Autodesk Inventor part; units mm, degrees
(part 2 of 4)
  spline S206 degree 2 poles (-53.4859, 25.985) (-53.3352, 26.0295) (-53.0931, 26.0739) (-52.9227, 26.0739) knots 0 0 0 1 2 2 2
  line L241 (-55.6274, 24.1399) -> (-55.6076, 24.1399)
  spline S207 degree 2 poles (-55.6076, 24.1399) (-55.5632, 24.1276) (-55.4668, 24.1226) (-55.4001, 24.1226) knots 0 0 0 1 2 2 2
  spline S208 degree 2 poles (-55.4001, 24.1226) (-55.2445, 24.1226) (-54.9382, 24.2585) (-54.7999, 24.3919) knots 0 0 0 1 2 2 2
  line L242 (-54.7999, 24.3919) -> (-54.7999, 26.0147)
  line L243 (-54.7999, 26.0147) -> (-54.4146, 26.0147)
  line L244 (-54.4146, 26.0147) -> (-54.4146, 23.7274)
  line L245 (-54.4146, 23.7274) -> (-54.7999, 23.7274)
  line L246 (-54.7999, 23.7274) -> (-54.7999, 24.0683)
  spline S209 degree 2 poles (-54.7999, 24.0683) (-55.0099, 23.8806) (-55.3236, 23.7274) (-55.4718, 23.7274) knots 0 0 0 1 2 2 2
  spline S210 degree 2 poles (-55.4718, 23.7274) (-55.5311, 23.7274) (-55.5903, 23.7324) (-55.6274, 23.7398) knots 0 0 0 1 2 2 2
  line L247 (-55.6274, 23.7398) -> (-55.6274, 24.1399)
  spline S211 degree 2 poles (-57.8059, 24.871) (-57.8059, 25.449) (-57.2502, 26.0789) (-56.7858, 26.0789) knots 0 0 0 1 2 2 2
  spline S212 degree 2 poles (-56.7858, 26.0789) (-56.3091, 26.0789) (-55.7632, 25.4293) (-55.7632, 24.871) knots 0 0 0 1 2 2 2
  spline S213 degree 2 poles (-55.7632, 24.871) (-55.7632, 24.298) (-56.3264, 23.6632) (-56.7858, 23.6632) knots 0 0 0 1 2 2 2
  spline S214 degree 2 poles (-56.7858, 23.6632) (-57.2502, 23.6632) (-57.8059, 24.2955) (-57.8059, 24.871) knots 0 0 0 1 2 2 2
  spline S215 degree 2 poles (-57.4083, 24.871) (-57.4083, 24.4264) (-57.0847, 23.9942) (-56.7858, 23.9942) knots 0 0 0 1 2 2 2
  spline S216 degree 2 poles (-56.7858, 23.9942) (-56.4869, 23.9942) (-56.1609, 24.4264) (-56.1609, 24.871) knots 0 0 0 1 2 2 2
  spline S217 degree 2 poles (-56.1609, 24.871) (-56.1609, 25.3033) (-56.4869, 25.7479) (-56.7858, 25.7479) knots 0 0 0 1 2 2 2
  spline S218 degree 2 poles (-56.7858, 25.7479) (-57.0822, 25.7479) (-57.4083, 25.3107) (-57.4083, 24.871) knots 0 0 0 1 2 2 2
  line L248 (-59.9795, 26.0147) -> (-59.5942, 26.0147)
  line L249 (-59.5942, 26.0147) -> (-59.5942, 25.7627)
  spline S219 degree 2 poles (-59.5942, 25.7627) (-59.4164, 25.9183) (-59.0978, 26.0789) (-58.9002, 26.0789) knots 0 0 0 1 2 2 2
  spline S220 degree 2 poles (-58.9002, 26.0789) (-58.752, 26.0789) (-58.4877, 25.9801) (-58.3913, 25.8739) knots 0 0 0 1 2 2 2
  spline S221 degree 2 poles (-58.3913, 25.8739) (-58.2925, 25.7677) (-58.1838, 25.4441) (-58.1838, 25.2119) knots 0 0 0 1 2 2 2
  line L250 (-58.1838, 25.2119) -> (-58.1838, 23.7274)
  line L251 (-58.1838, 23.7274) -> (-58.5692, 23.7274)
  line L252 (-58.5692, 23.7274) -> (-58.5692, 25.0316)
  spline S222 degree 2 poles (-58.5692, 25.0316) (-58.5692, 25.2144) (-58.5963, 25.454) (-58.6433, 25.5429) knots 0 0 0 1 2 2 2
  spline S223 degree 2 poles (-58.6433, 25.5429) (-58.6902, 25.6318) (-58.8508, 25.7133) (-59.0014, 25.7133) knots 0 0 0 1 2 2 2
  spline S224 degree 2 poles (-59.0014, 25.7133) (-59.1422, 25.7133) (-59.4608, 25.5528) (-59.5942, 25.4367) knots 0 0 0 1 2 2 2
  line L253 (-59.5942, 25.4367) -> (-59.5942, 23.7274)
  line L254 (-59.5942, 23.7274) -> (-59.9795, 23.7274)
  line L255 (-59.9795, 23.7274) -> (-59.9795, 26.0147)
  line L256 (-62.3335, 26.0147) -> (-61.9482, 26.0147)
  line L257 (-61.9482, 26.0147) -> (-61.9482, 24.7105)
  spline S225 degree 2 poles (-61.9482, 24.7105) (-61.9482, 24.5524) (-61.9185, 24.2807) (-61.8741, 24.1992) knots 0 0 0 1 2 2 2
  spline S226 degree 2 poles (-61.8741, 24.1992) (-61.8271, 24.1127) (-61.6592, 24.0288) (-61.5159, 24.0288) knots 0 0 0 1 2 2 2
  spline S227 degree 2 poles (-61.5159, 24.0288) (-61.3726, 24.0288) (-61.0688, 24.1819) (-60.9231, 24.3054) knots 0 0 0 1 2 2 2
  line L258 (-60.9231, 24.3054) -> (-60.9231, 26.0147)
  line L259 (-60.9231, 26.0147) -> (-60.5378, 26.0147)
  line L260 (-60.5378, 26.0147) -> (-60.5378, 23.7274)
  line L261 (-60.5378, 23.7274) -> (-60.9231, 23.7274)
  line L262 (-60.9231, 23.7274) -> (-60.9231, 23.9818)
  spline S228 degree 2 poles (-60.9231, 23.9818) (-61.096, 23.8262) (-61.4294, 23.6632) (-61.6172, 23.6632) knots 0 0 0 1 2 2 2
  spline S229 degree 2 poles (-61.6172, 23.6632) (-61.9531, 23.6632) (-62.3335, 24.1078) (-62.3335, 24.5302) knots 0 0 0 1 2 2 2
  line L263 (-62.3335, 24.5302) -> (-62.3335, 26.0147)
  line L264 (-64.6331, 26.0147) -> (-64.2477, 26.0147)
  line L265 (-64.2477, 26.0147) -> (-64.2477, 25.7825)
  spline S230 degree 2 poles (-64.2477, 25.7825) (-64.1588, 25.8566) (-64.0279, 25.9554) (-63.939, 25.9974) knots 0 0 0 1 2 2 2
  spline S231 degree 2 poles (-63.939, 25.9974) (-63.8575, 26.0369) (-63.6821, 26.0789) (-63.566, 26.0789) knots 0 0 0 1 2 2 2
  spline S232 degree 2 poles (-63.566, 26.0789) (-63.3783, 26.0789) (-63.0621, 25.9233) (-62.951, 25.7726) knots 0 0 0 1 2 2 2
  spline S233 degree 2 poles (-62.951, 25.7726) (-62.8398, 25.6219) (-62.7163, 25.1773) (-62.7163, 24.8883) knots 0 0 0 1 2 2 2
  spline S234 degree 2 poles (-62.7163, 24.8883) (-62.7163, 24.587) (-62.8719, 24.1473) (-63.0078, 23.9818) knots 0 0 0 1 2 2 2
  spline S235 degree 2 poles (-63.0078, 23.9818) (-63.1338, 23.8336) (-63.487, 23.6632) (-63.6821, 23.6632) knots 0 0 0 1 2 2 2
  spline S236 degree 2 poles (-63.6821, 23.6632) (-63.8525, 23.6632) (-64.1069, 23.7398) (-64.2477, 23.8188) knots 0 0 0 1 2 2 2
  line L266 (-64.2477, 23.8188) -> (-64.2477, 22.8308)
  line L267 (-64.2477, 22.8308) -> (-64.6331, 22.8308)
  line L268 (-64.6331, 22.8308) -> (-64.6331, 26.0147)
  line L269 (-64.2477, 25.4589) -> (-64.2477, 24.1374)
  spline S237 degree 2 poles (-64.2477, 24.1374) (-64.1045, 24.0683) (-63.8772, 24.0164) (-63.7463, 24.0164) knots 0 0 0 1 2 2 2
  spline S238 degree 2 poles (-63.7463, 24.0164) (-63.4499, 24.0164) (-63.114, 24.461) (-63.114, 24.8809) knots 0 0 0 1 2 2 2
  spline S239 degree 2 poles (-63.114, 24.8809) (-63.114, 25.286) (-63.3709, 25.7133) (-63.6549, 25.7133) knots 0 0 0 1 2 2 2
  spline S240 degree 2 poles (-63.6549, 25.7133) (-63.8056, 25.7133) (-64.1119, 25.575) (-64.2477, 25.4589) knots 0 0 0 1 2 2 2
  spline S241 degree 2 poles (51.1339, 19.6673) (51.5277, 19.8947) (52.3044, 19.9435) (52.6446, 19.8089) knots 0 0 0 1 2 2 2
  spline S242 degree 2 poles (52.6446, 19.8089) (53.0488, 19.6427) (53.6387, 19.0757) (53.9502, 18.5363) knots 0 0 0 1 2 2 2
  line L270 (53.9502, 18.5363) -> (54.8251, 17.0208)
  line L271 (54.8251, 17.0208) -> (49.5424, 13.9708)
  line L272 (49.5424, 13.9708) -> (48.7342, 15.3707)
  spline S243 degree 2 poles (48.7342, 15.3707) (48.4079, 15.9358) (48.1544, 16.5429) (48.1474, 16.8814) knots 0 0 0 1 2 2 2
  spline S244 degree 2 poles (48.1474, 16.8814) (48.1316, 17.2547) (48.4732, 17.8001) (48.8071, 17.9929) knots 0 0 0 1 2 2 2
  spline S245 degree 2 poles (48.8071, 17.9929) (49.1795, 18.2079) (49.9977, 18.1551) (50.3649, 17.9048) knots 0 0 0 1 2 2 2
  line L273 (50.3649, 17.9048) -> (50.3906, 17.9196)
  spline S246 degree 2 poles (50.3906, 17.9196) (50.2471, 18.4646) (50.6287, 19.3756) (51.1339, 19.6673) knots 0 0 0 1 2 2 2
  spline S247 degree 2 poles (51.5865, 18.9525) (51.2868, 18.7795) (51.0004, 18.3858) (51.0117, 18.0499) knots 0 0 0 1 2 2 2
  spline S248 degree 2 poles (51.0117, 18.0499) (51.0225, 17.8335) (51.1985, 17.41) (51.4086, 17.0461) knots 0 0 0 1 2 2 2
  line L274 (51.4086, 17.0461) -> (51.8683, 16.2498)
  line L275 (51.8683, 16.2498) -> (53.8204, 17.3769)
  line L276 (53.8204, 17.3769) -> (53.4917, 17.9463)
  spline S249 degree 2 poles (53.4917, 17.9463) (53.2248, 18.4086) (52.8327, 18.89) (52.577, 19.0164) knots 0 0 0 1 2 2 2
  spline S250 degree 2 poles (52.577, 19.0164) (52.3221, 19.1318) (51.8648, 19.1132) (51.5865, 18.9525) knots 0 0 0 1 2 2 2
  spline S251 degree 2 poles (49.3282, 17.3177) (49.1398, 17.2089) (48.9314, 16.9173) (48.9317, 16.7291) knots 0 0 0 1 2 2 2
  spline S252 degree 2 poles (48.9317, 16.7291) (48.9364, 16.5035) (49.1333, 16.0635) (49.3483, 15.6911) knots 0 0 0 1 2 2 2
  line L277 (49.3483, 15.6911) -> (49.7364, 15.019)
  line L278 (49.7364, 15.019) -> (51.2818, 15.9112)
  line L279 (51.2818, 15.9112) -> (50.8221, 16.7075)
  spline S253 degree 2 poles (50.8221, 16.7075) (50.6318, 17.0371) (50.3828, 17.3101) (50.1794, 17.4153) knots 0 0 0 1 2 2 2
  spline S254 degree 2 poles (50.1794, 17.4153) (49.9828, 17.5186) (49.5765, 17.461) (49.3282, 17.3177) knots 0 0 0 1 2 2 2
  spline S255 degree 2 poles (50.6883, 23.2173) (50.7951, 23.1705) (51.1674, 23.0201) (51.3057, 22.9288) knots 0 0 0 1 2 2 2
  spline S256 degree 2 poles (51.3057, 22.9288) (51.5013, 22.8076) (51.79, 22.5348) (51.9631, 22.2352) knots 0 0 0 1 2 2 2
  spline S257 degree 2 poles (51.9631, 22.2352) (52.1039, 21.9911) (52.1744, 21.4439) (52.1039, 21.1806) knots 0 0 0 1 2 2 2
  spline S258 degree 2 poles (52.1039, 21.1806) (52.0326, 20.9282) (51.6644, 20.4588) (51.399, 20.3055) knots 0 0 0 1 2 2 2
  spline S259 degree 2 poles (51.399, 20.3055) (50.988, 20.0683) (50.2056, 20.0789) (49.8211, 20.3592) knots 0 0 0 1 2 2 2
  spline S260 degree 2 poles (49.8211, 20.3592) (49.4742, 20.6041) (48.8346, 21.445) (48.5007, 21.9542) knots 0 0 0 1 2 2 2
  line L280 (48.5007, 21.9542) -> (48.3722, 21.8801)
  spline S261 degree 2 poles (48.3722, 21.8801) (48.1411, 21.7466) (47.9358, 21.4398) (47.9286, 21.2644) knots 0 0 0 1 2 2 2
  spline S262 degree 2 poles (47.9286, 21.2644) (47.9214, 21.089) (48.0826, 20.6911) (48.1963, 20.4942) knots 0 0 0 1 2 2 2
  spline S263 degree 2 poles (48.1963, 20.4942) (48.3298, 20.263) (48.8276, 19.7171) (49.1408, 19.4812) knots 0 0 0 1 2 2 2
  line L281 (49.1408, 19.4812) -> (49.163, 19.4427)
  line L282 (49.163, 19.4427) -> (48.4823, 19.0497)
  spline S264 degree 2 poles (48.4823, 19.0497) (48.3247, 19.2041) (47.7983, 19.8192) (47.603, 20.1574) knots 0 0 0 1 2 2 2
  spline S265 degree 2 poles (47.603, 20.1574) (47.3658, 20.5684) (47.1704, 21.2034) (47.2089, 21.5224) knots 0 0 0 1 2 2 2
  spline S266 degree 2 poles (47.2089, 21.5224) (47.2455, 21.8346) (47.6399, 22.3477) (48.0123, 22.5628) knots 0 0 0 1 2 2 2
  line L283 (48.0123, 22.5628) -> (50.7222, 24.1273)
  line L284 (50.7222, 24.1273) -> (51.1078, 23.4595)
  line L285 (51.1078, 23.4595) -> (50.6883, 23.2173)
  line L286 (50.1317, 22.8959) -> (49.0315, 22.2607)
  spline S267 degree 2 poles (49.0315, 22.2607) (49.1913, 22.0333) (49.6818, 21.3519) (49.8813, 21.1645) knots 0 0 0 1 2 2 2
  spline S268 degree 2 poles (49.8813, 21.1645) (50.1159, 20.9461) (50.6543, 20.7946) (50.954, 20.9676) knots 0 0 0 1 2 2 2
  spline S269 degree 2 poles (50.954, 20.9676) (51.2964, 21.1653) (51.4207, 21.7508) (51.2082, 22.119) knots 0 0 0 1 2 2 2
  spline S270 degree 2 poles (51.2082, 22.119) (51.0278, 22.4315) (50.4615, 22.7895) (50.1317, 22.8959) knots 0 0 0 1 2 2 2
  spline S271 degree 2 poles (49.5659, 26.308) (49.8798, 25.7643) (49.6125, 24.7938) (48.9404, 24.4057) knots 0 0 0 1 2 2 2
  line L287 (48.9404, 24.4057) -> (46.7443, 23.1378)
  line L288 (46.7443, 23.1378) -> (47.0038, 22.6883)
  line L289 (47.0038, 22.6883) -> (46.4515, 22.3694)
  line L290 (46.4515, 22.3694) -> (46.192, 22.8189)
  line L291 (46.192, 22.8189) -> (45.0533, 22.1615)
  line L292 (45.0533, 22.1615) -> (44.6677, 22.8293)
  line L293 (44.6677, 22.8293) -> (45.8064, 23.4868)
  line L294 (45.8064, 23.4868) -> (45.0971, 24.7154)
  line L295 (45.0971, 24.7154) -> (45.6493, 25.0342)
  line L296 (45.6493, 25.0342) -> (46.3587, 23.8056)
  line L297 (46.3587, 23.8056) -> (48.2466, 24.8956)
  spline S272 degree 2 poles (48.2466, 24.8956) (48.5463, 25.0686) (48.8635, 25.2803) (48.9628, 25.4347) knots 0 0 0 1 2 2 2
  spline S273 degree 2 poles (48.9628, 25.4347) (49.0523, 25.5663) (49.0208, 25.9077) (48.8873, 26.1388) knots 0 0 0 1 2 2 2
  spline S274 degree 2 poles (48.8873, 26.1388) (48.7934, 26.3015) (48.5194, 26.5486) (48.4499, 26.5998) knots 0 0 0 1 2 2 2
  line L298 (48.4499, 26.5998) -> (48.4277, 26.6383)
  line L299 (48.4277, 26.6383) -> (49.027, 26.9844)
  spline S275 degree 2 poles (49.027, 26.9844) (49.1872, 26.8257) (49.4695, 26.475) (49.5659, 26.308) knots 0 0 0 1 2 2 2
  spline S276 degree 2 poles (48.162, 28.7396) (48.4759, 28.1959) (48.2086, 27.2254) (47.5365, 26.8373) knots 0 0 0 1 2 2 2
  line L300 (47.5365, 26.8373) -> (45.3404, 25.5694)
  line L301 (45.3404, 25.5694) -> (45.5999, 25.1199)
  line L302 (45.5999, 25.1199) -> (45.0476, 24.801)
  line L303 (45.0476, 24.801) -> (44.7881, 25.2505)
  line L304 (44.7881, 25.2505) -> (43.6494, 24.5931)
  line L305 (43.6494, 24.5931) -> (43.2638, 25.2609)
  line L306 (43.2638, 25.2609) -> (44.4025, 25.9184)
  line L307 (44.4025, 25.9184) -> (43.6932, 27.147)
  line L308 (43.6932, 27.147) -> (44.2454, 27.4659)
  line L309 (44.2454, 27.4659) -> (44.9548, 26.2372)
  line L310 (44.9548, 26.2372) -> (46.8427, 27.3272)
  spline S277 degree 2 poles (46.8427, 27.3272) (47.1424, 27.5002) (47.4597, 27.7119) (47.5589, 27.8663) knots 0 0 0 1 2 2 2
  spline S278 degree 2 poles (47.5589, 27.8663) (47.6485, 27.9979) (47.6169, 28.3393) (47.4834, 28.5704) knots 0 0 0 1 2 2 2
  spline S279 degree 2 poles (47.4834, 28.5704) (47.3895, 28.7331) (47.1156, 28.9802) (47.046, 29.0314) knots 0 0 0 1 2 2 2
  line L311 (47.046, 29.0314) -> (47.0238, 29.0699)
  line L312 (47.0238, 29.0699) -> (47.6231, 29.416)
  spline S280 degree 2 poles (47.6231, 29.416) (47.7833, 29.2573) (48.0656, 28.9066) (48.162, 28.7396) knots 0 0 0 1 2 2 2
  spline S281 degree 2 poles (46.4695, 31.7009) (47.0182, 30.7505) (46.5553, 29.0905) (45.5706, 28.5221) knots 0 0 0 1 2 2 2
  spline S282 degree 2 poles (45.5706, 28.5221) (44.6031, 27.9635) (42.87, 28.3157) (42.398, 29.1333) knots 0 0 0 1 2 2 2
  spline S283 degree 2 poles (42.398, 29.1333) (42.1854, 29.5015) (42.0707, 30.1945) (42.1765, 30.5352) knots 0 0 0 1 2 2 2
  spline S284 degree 2 poles (42.1765, 30.5352) (42.2798, 30.8803) (42.8038, 31.4853) (43.279, 31.7597) knots 0 0 0 1 2 2 2
  line L313 (43.279, 31.7597) -> (43.6429, 31.9698)
  line L314 (43.6429, 31.9698) -> (45.2272, 29.2257)
  spline S285 degree 2 poles (45.2272, 29.2257) (45.9164, 29.6236) (46.2481, 30.7398) (45.8922, 31.3562) knots 0 0 0 1 2 2 2
  spline S286 degree 2 poles (45.8922, 31.3562) (45.7661, 31.5746) (45.423, 31.9415) (45.247, 32.0683) knots 0 0 0 1 2 2 2
  spline S287 degree 2 poles (45.247, 32.0683) (45.0576, 32.1986) (44.7644, 32.3604) (44.649, 32.4022) knots 0 0 0 1 2 2 2
  line L315 (44.649, 32.4022) -> (44.6267, 32.4408)
  line L316 (44.6267, 32.4408) -> (45.3545, 32.8609)
  spline S288 degree 2 poles (45.3545, 32.8609) (45.4683, 32.7725) (45.808, 32.5006) (45.9256, 32.3858) knots 0 0 0 1 2 2 2
  spline S289 degree 2 poles (45.9256, 32.3858) (46.0925, 32.2253) (46.331, 31.9407) (46.4695, 31.7009) knots 0 0 0 1 2 2 2
  spline S290 degree 2 poles (43.5091, 31.0249) (43.2444, 30.8607) (42.9148, 30.522) (42.8439, 30.3383) knots 0 0 0 1 2 2 2
  spline S291 degree 2 poles (42.8439, 30.3383) (42.7608, 30.1362) (42.8125, 29.6809) (42.9682, 29.4112) knots 0 0 0 1 2 2 2
  spline S292 degree 2 poles (42.9682, 29.4112) (43.1214, 29.1458) (43.4948, 28.8648) (43.7379, 28.7996) knots 0 0 0 1 2 2 2
  spline S293 degree 2 poles (43.7379, 28.7996) (43.9828, 28.7412) (44.4528, 28.8071) (44.7178, 28.9315) knots 0 0 0 1 2 2 2
  line L317 (44.7178, 28.9315) -> (43.5091, 31.0249)
  line L318 (40.7031, 33.977) -> (40.7229, 33.9427)
  spline S294 degree 2 poles (40.7229, 33.9427) (40.746, 33.8533) (40.8338, 33.6814) (40.9005, 33.5658) knots 0 0 0 1 2 2 2
  spline S295 degree 2 poles (40.9005, 33.5658) (41.0563, 33.2961) (41.5982, 32.9012) (41.9678, 32.795) knots 0 0 0 1 2 2 2
  line L319 (41.9678, 32.795) -> (44.7804, 34.4188)
  line L320 (44.7804, 34.4188) -> (45.166, 33.751)
  line L321 (45.166, 33.751) -> (41.2018, 31.4623)
  line L322 (41.2018, 31.4623) -> (40.8162, 32.1301)
  line L323 (40.8162, 32.1301) -> (41.407, 32.4712)
  spline S296 degree 2 poles (41.407, 32.4712) (40.8715, 32.6472) (40.2922, 33.0377) (40.1439, 33.2945) knots 0 0 0 1 2 2 2
  spline S297 degree 2 poles (40.1439, 33.2945) (40.0846, 33.3973) (40.0338, 33.505) (40.0096, 33.5766) knots 0 0 0 1 2 2 2
  line L324 (40.0096, 33.5766) -> (40.7031, 33.977)
  line L325 (37.8922, 37.1945) -> (44.5472, 38.1941)
  line L326 (44.5472, 38.1941) -> (44.9599, 37.4792)
  line L327 (44.9599, 37.4792) -> (42.8972, 37.2358)
  line L328 (42.8972, 37.2358) -> (39.9561, 33.6199)
  line L329 (39.9561, 33.6199) -> (39.5408, 34.3391)
  line L330 (39.5408, 34.3391) -> (41.8523, 37.1177)
  line L331 (41.8523, 37.1177) -> (38.2927, 36.501)
  line L332 (38.2927, 36.501) -> (37.8922, 37.1945)
  line L333 (-3.1702, 31) -> (2.684, 31)
  line L334 (2.684, 31) -> (2.684, 32.2253)
  line L335 (2.684, 32.2253) -> (0.5057, 32.2253)
  line L336 (0.5057, 32.2253) -> (0.5057, 40.2674)
  line L337 (0.5057, 40.2674) -> (2.684, 40.2674)
  line L338 (2.684, 40.2674) -> (2.684, 41.3663)
  spline S298 degree 2 poles (2.684, 41.3663) (1.4489, 41.3663) (0.282, 42.0665) (0.2042, 43.0389) knots 0 0 0 1 2 2 2
  line L339 (0.2042, 43.0389) -> (-1.0405, 43.0389)
  line L340 (-1.0405, 43.0389) -> (-1.0405, 32.2253)
  line L341 (-1.0405, 32.2253) -> (-3.1702, 32.2253)
  line L342 (-3.1702, 32.2253) -> (-3.1702, 31)
  dimension "d46" = 6
  dimension "d47" = 6
  dimension "d48" = 73.2452
  dimension "d49" = 32.174
  dimension "d50" = 25
  dimension "d51" = 25
  constraints: 62 end point, 15 parallel, 9 horizontal, 7 perpendicular, 1 point on line, 1 vertical, 3 other
  measures "d46" distance of L5.end L6.end
  measures "d47" distance of L10.end L9.end
  measures "d48" distance between parallel lines of L2 L6
  measures "d49" distance of L13.start L12.end
  measures "d50" distance of L16.end L15.end
  measures "d51" distance of L15.end L14.end
emboss "Emboss1" sketch "Sketch6" operation cut depth 1 direction (0, -1, 0)
sketch "Sketch7" plane through (0, 10, 0) normal (0, 1, 0) x (1, 0, 0)
  line L0 (0.5057, 40.2674) -> (2.684, 40.2674) projected
  line L1 (2.684, 40.2674) -> (2.684, 41.3663) projected
  line L2 (0.2042, 43.0389) -> (-1.0405, 43.0389) projected
  line L3 (-1.0405, 43.0389) -> (-1.0405, 32.2253) projected
  line L4 (-1.0405, 32.2253) -> (-3.1702, 32.2253) projected
  line L5 (-3.1702, 32.2253) -> (-3.1702, 31) projected
  line L6 (-3.1702, 31) -> (2.684, 31) projected
  line L7 (2.684, 31) -> (2.684, 32.2253) projected
  line L8 (2.684, 32.2253) -> (0.5057, 32.2253) projected
  line L9 (0.5057, 32.2253) -> (0.5057, 40.2674) projected
  line L10 (11.4709, -68.4771) -> (10.6948, -68.4771) projected
  line L11 (10.6948, -68.4771) -> (10.6948, -69.1) projected
  line L12 (10.6948, -69.1) -> (13.0577, -69.1) projected
  line L13 (13.0577, -69.1) -> (13.0577, -68.4771) projected
  line L14 (13.0577, -68.4771) -> (12.2816, -68.4771) projected
  line L15 (12.2816, -68.4771) -> (12.2816, -63.6229) projected
  line L16 (12.2816, -63.6229) -> (13.0577, -63.6229) projected
  line L17 (13.0577, -63.6229) -> (13.0577, -63) projected
  line L18 (13.0577, -63) -> (10.6948, -63) projected
  line L19 (10.6948, -63) -> (10.6948, -63.6229) projected
  line L20 (10.6948, -63.6229) -> (11.4709, -63.6229) projected
  line L21 (11.4709, -63.6229) -> (11.4709, -68.4771) projected
  line L22 (17.4473, -69.1) -> (17.4473, -63) projected
  line L23 (17.4473, -63) -> (16.6366, -63) projected
  line L24 (16.6366, -63) -> (16.6366, -65.2739) projected
  line L25 (16.6366, -65.2739) -> (15.9495, -65.2739) projected
  line L26 (15.9149, -69.1) -> (17.4473, -69.1) projected
  line L27 (16.0829, -65.966) -> (16.6366, -65.966) projected
  line L28 (16.6366, -65.966) -> (16.6366, -68.3981) projected
  line L29 (16.6366, -68.3981) -> (15.9643, -68.3981) projected
  line L30 (-5.2028, -67.8444) -> (-5.2621, -67.8444) projected
  line L31 (-5.2621, -67.8444) -> (-5.2621, -68.8133) projected
  line L32 (-1.4113, -64.3841) -> (-1.352, -64.3841) projected
  line L33 (-1.352, -64.3841) -> (-1.352, -63.3658) projected
  line L34 (21.0806, -69.1) -> (22.6526, -69.1) projected
  line L35 (22.6526, -69.1) -> (22.6526, -63) projected
  line L36 (22.6526, -63) -> (21.8419, -63) projected
  line L37 (21.8419, -63) -> (21.8419, -65.4271) projected
  line L38 (21.8419, -65.4271) -> (20.9125, -65.4271) projected
  line L39 (20.9125, -65.4271) -> (18.9846, -63) projected
  line L40 (18.9846, -63) -> (17.9317, -63) projected
  line L41 (17.9317, -63) -> (20.1018, -65.6545) projected
  line L42 (21.13, -66.1044) -> (21.8419, -66.1044) projected
  line L43 (21.8419, -66.1044) -> (21.8419, -68.3981) projected
  line L44 (21.8419, -68.3981) -> (21.0361, -68.3981) projected
  line L45 (-10.9568, -63) -> (-11.7279, -63) projected
  line L46 (-11.7279, -63) -> (-11.7279, -67.5775) projected
  line L47 (-11.7279, -67.5775) -> (-10.9568, -67.5775) projected
  line L48 (-10.9568, -67.5775) -> (-10.9568, -63) projected
  line L49 (-15.7419, -65.7979) -> (-13.3246, -65.7979) projected
  line L50 (-13.3246, -65.2096) -> (-16.4932, -65.2096) projected
  line L51 (-16.4932, -65.2096) -> (-16.4932, -65.6298) projected
  line L52 (-16.4092, -63.2818) -> (-16.4092, -64.1221) projected
  line L53 (-16.4092, -64.1221) -> (-16.3647, -64.1221) projected
  line L54 (4.9754, -68.0669) -> (4.9754, -66.0006) projected
  line L55 (4.9754, -66.0006) -> (7.0417, -66.0006) projected
  line L56 (7.0417, -66.0006) -> (7.0417, -65.3431) projected
  line L57 (7.0417, -65.3431) -> (4.9754, -65.3431) projected
  line L58 (4.9754, -65.3431) -> (4.9754, -63.2768) projected
  line L59 (4.9754, -63.2768) -> (4.2932, -63.2768) projected
  line L60 (4.2932, -63.2768) -> (4.2932, -65.3431) projected
  line L61 (4.2932, -65.3431) -> (2.2269, -65.3431) projected
  line L62 (2.2269, -65.3431) -> (2.2269, -66.0006) projected
  line L63 (2.2269, -66.0006) -> (4.2932, -66.0006) projected
  line L64 (4.2932, -66.0006) -> (4.2932, -68.0669) projected
  line L65 (4.2932, -68.0669) -> (4.9754, -68.0669) projected
  line L66 (-17.2891, -63) -> (-18.0603, -63) projected
  line L67 (-18.0603, -63) -> (-18.0603, -69.3719) projected
  line L68 (-18.0603, -69.3719) -> (-17.2891, -69.3719) projected
  line L69 (-17.2891, -69.3719) -> (-17.2891, -63) projected
  line L70 (-6.2656, -69.3719) -> (-6.2656, -63) projected
  line L71 (-6.2656, -63) -> (-7.0368, -63) projected
  line L72 (-7.0368, -63) -> (-7.0368, -66.4207) projected
  line L73 (-9.0882, -65.61) -> (-9.0882, -63) projected
  line L74 (-9.0882, -63) -> (-9.8594, -63) projected
  line L75 (-9.8594, -63) -> (-9.8594, -65.9709) projected
  line L76 (-7.0368, -67.0683) -> (-7.0368, -69.3719) projected
  line L77 (-7.0368, -69.3719) -> (-6.2656, -69.3719) projected
  line L78 (-34.4486, 9.7771) -> (-34.4486, 9.2238) projected
  line L79 (-34.4486, 9.2238) -> (-31.4006, 9.2238) projected
  line L80 (-31.4006, 9.2238) -> (-31.4006, 9.6017) projected
  line L81 (-31.4006, 9.6017) -> (-34.0263, 9.6017) projected
  line L82 (-34.0263, 9.6017) -> (-32.2404, 10.3897) projected
  line L83 (-32.2404, 10.3897) -> (-32.2404, 10.6367) projected
  line L84 (-32.2404, 10.6367) -> (-34.0263, 11.432) projected
  line L85 (-34.0263, 11.432) -> (-31.4006, 11.432) projected
  line L86 (-31.4006, 11.432) -> (-31.4006, 11.8371) projected
  line L87 (-31.4006, 11.8371) -> (-34.4486, 11.8371) projected
  line L88 (-34.4486, 11.8371) -> (-34.4486, 11.2739) projected
  line L89 (-34.4486, 11.2739) -> (-32.7517, 10.5379) projected
  line L90 (-32.7517, 10.5379) -> (-34.4486, 9.7771) projected
  line L91 (-11.7823, -68.3387) -> (-11.7823, -69.1395) projected
  line L92 (-11.7823, -69.1395) -> (-10.9073, -69.1395) projected
  line L93 (-10.9073, -69.1395) -> (-10.9073, -68.3387) projected
  line L94 (-10.9073, -68.3387) -> (-11.7823, -68.3387) projected
  line L95 (-31.4006, 14.769) -> (-31.4006, 15.1543) projected
  line L96 (-31.4006, 15.1543) -> (-34.5845, 15.1543) projected
  line L97 (-34.5845, 15.1543) -> (-34.5845, 14.769) projected
  line L98 (-34.5845, 14.769) -> (-31.4006, 14.769) projected
  line L99 (-21.9407, -63.4647) -> (-21.9407, -63) projected
  line L100 (-21.9407, -63) -> (-22.7119, -63) projected
  line L101 (-22.7119, -63) -> (-22.7119, -69.3719) projected
  line L102 (-22.7119, -69.3719) -> (-21.9407, -69.3719) projected
  line L103 (-21.9407, -69.3719) -> (-21.9407, -67.3946) projected
  line L104 (-21.9407, -66.7569) -> (-21.9407, -64.1122) projected
  line L105 (-31.4006, 17.1303) -> (-31.4006, 17.5157) projected
  line L106 (-31.4006, 17.5157) -> (-33.6879, 17.5157) projected
  line L107 (-33.6879, 17.5157) -> (-33.6879, 17.1303) projected
  line L108 (-33.6879, 17.1303) -> (-31.4006, 17.1303) projected
  line L109 (-35.1477, -24.1889) -> (-33.6654, -23.3332) projected
  line L110 (-33.6654, -23.3332) -> (-33.7092, -23.2574) projected
  line L111 (-26.507, -19.4922) -> (-25.0332, -18.6413) projected
  line L112 (-25.0332, -18.6413) -> (-28.7333, -12.2324) projected
  line L113 (-28.7333, -12.2324) -> (-29.9376, -12.9277) projected
  line L114 (-29.9376, -12.9277) -> (-26.9911, -18.0312) projected
  line L115 (-31.8279, 18.4666) -> (-33.1272, 18.4666) projected
  line L116 (-33.4483, 18.4666) -> (-33.6879, 18.4666) projected
  line L117 (-33.6879, 18.4666) -> (-33.6879, 18.0813) projected
  line L118 (-33.6879, 18.0813) -> (-30.5584, 18.0813) projected
  line L119 (-30.5584, 18.0813) -> (-30.5584, 18.4666) projected
  line L120 (-30.5584, 18.4666) -> (-31.5167, 18.4666) projected
  line L121 (-32.3837, 12.793) -> (-33.6879, 12.793) projected
  line L122 (-33.6879, 12.793) -> (-33.6879, 12.4077) projected
  line L123 (-33.6879, 12.4077) -> (-32.2034, 12.4077) projected
  line L124 (-31.6526, 13.818) -> (-31.4006, 13.818) projected
  line L125 (-31.4006, 13.818) -> (-31.4006, 14.2034) projected
  line L126 (-31.4006, 14.2034) -> (-33.6879, 14.2034) projected
  line L127 (-33.6879, 14.2034) -> (-33.6879, 13.818) projected
  line L128 (-33.6879, 13.818) -> (-31.9786, 13.818) projected
  line L129 (-31.4006, 20.4056) -> (-31.4006, 20.7909) projected
  line L130 (-31.4006, 20.7909) -> (-34.5845, 20.7909) projected
  line L131 (-34.5845, 20.7909) -> (-34.5845, 20.4056) projected
  line L132 (-34.5845, 20.4056) -> (-31.4006, 20.4056) projected
  line L133 (-33.3692, 16.13) -> (-33.3692, 16.8389) projected
  line L134 (-33.3692, 16.8389) -> (-33.6879, 16.8389) projected
  line L135 (-33.6879, 16.8389) -> (-33.6879, 16.13) projected
  line L136 (-33.6879, 16.13) -> (-34.3449, 16.13) projected
  line L137 (-34.3449, 16.13) -> (-34.3449, 15.7446) projected
  line L138 (-34.3449, 15.7446) -> (-33.6879, 15.7446) projected
  line L139 (-33.6879, 15.7446) -> (-33.6879, 15.4853) projected
  line L140 (-33.6879, 15.4853) -> (-33.3692, 15.4853) projected
  line L141 (-33.3692, 15.4853) -> (-33.3692, 15.7446) projected
  line L142 (-33.3692, 15.7446) -> (-32.1021, 15.7446) projected
  line L143 (-31.4204, 16.8389) -> (-31.7662, 16.8389) projected
  line L144 (-31.7662, 16.8389) -> (-31.7662, 16.8166) projected
  line L145 (-32.28, 16.13) -> (-33.3692, 16.13) projected
  line L146 (-32.7987, 27.0771) -> (-32.7987, 25.8692) projected
  line L147 (-32.5047, 25.8692) -> (-32.5047, 27.4525) projected
  line L148 (-32.5047, 27.4525) -> (-32.7147, 27.4525) projected
  line L149 (-31.5414, 27.4105) -> (-31.9613, 27.4105) projected
  line L150 (-31.9613, 27.4105) -> (-31.9613, 27.3883) projected
  line L151 (-34.0683, 17.5428) -> (-34.4684, 17.5428) projected
  line L152 (-34.4684, 17.5428) -> (-34.4684, 17.1056) projected
  line L153 (-34.4684, 17.1056) -> (-34.0683, 17.1056) projected
  line L154 (-34.0683, 17.1056) -> (-34.0683, 17.5428) projected
  line L155 (-33.347, 28.2281) -> (-33.6879, 28.2281) projected
  line L156 (-33.6879, 28.2281) -> (-33.6879, 27.8428) projected
  line L157 (-33.6879, 27.8428) -> (-31.4006, 27.8428) projected
  line L158 (-31.4006, 27.8428) -> (-31.4006, 28.2281) projected
  line L159 (-31.4006, 28.2281) -> (-33.0234, 28.2281) projected
  line L160 (-33.2754, 29.0358) -> (-33.2754, 29.0556) projected
  line L161 (-33.2754, 29.0556) -> (-33.6755, 29.0556) projected
  line L162 (-32.5047, 21.5887) -> (-32.5047, 23.172) projected
  line L163 (-32.5047, 23.172) -> (-32.7147, 23.172) projected
  line L164 (-31.5414, 23.13) -> (-31.9613, 23.13) projected
  line L165 (-31.9613, 23.13) -> (-31.9613, 23.1078) projected
  line L166 (-32.7987, 22.7965) -> (-32.7987, 21.5887) projected
  line L167 (-32.8357, 24.3354) -> (-33.6879, 23.7821) projected
  line L168 (-33.6879, 23.7821) -> (-33.6879, 23.3103) projected
  line L169 (-33.6879, 23.3103) -> (-32.5344, 24.0958) projected
  line L170 (-32.5344, 24.0958) -> (-31.4006, 23.3029) projected
  line L171 (-31.4006, 23.3029) -> (-31.4006, 23.7401) projected
  line L172 (-31.4006, 23.7401) -> (-32.2602, 24.3107) projected
  line L173 (-32.2602, 24.3107) -> (-31.4006, 24.8664) projected
  line L174 (-31.4006, 24.8664) -> (-31.4006, 25.3382) projected
  line L175 (-31.4006, 25.3382) -> (-32.5591, 24.5503) projected
  line L176 (-32.5591, 24.5503) -> (-33.6879, 25.3382) projected
  line L177 (-33.6879, 25.3382) -> (-33.6879, 24.901) projected
  line L178 (-33.6879, 24.901) -> (-32.8357, 24.3354) projected
  line L179 (-54.9741, 18.6224) -> (-54.9741, 20.9097) projected
  line L180 (-54.9741, 20.9097) -> (-55.3594, 20.9097) projected
  line L181 (-55.3594, 20.9097) -> (-55.3594, 19.2004) projected
  line L182 (-56.2708, 19.5858) -> (-56.2708, 20.9097) projected
  line L183 (-56.2708, 20.9097) -> (-56.6561, 20.9097) projected
  line L184 (-56.6561, 20.9097) -> (-56.6561, 19.403) projected
  line L185 (-57.5676, 19.5858) -> (-57.5676, 20.9097) projected
  line L186 (-57.5676, 20.9097) -> (-57.9529, 20.9097) projected
  line L187 (-57.9529, 20.9097) -> (-57.9529, 19.403) projected
  line L188 (-55.3594, 18.8744) -> (-55.3594, 18.6224) projected
  line L189 (-55.3594, 18.6224) -> (-54.9741, 18.6224) projected
  line L190 (-52.3188, 18.5533) -> (-52.3509, 18.5533) projected
  line L191 (-52.3509, 18.5533) -> (-52.3509, 18.0642) projected
  line L192 (-52.3509, 20.7022) -> (-52.3509, 20.2181) projected
  line L193 (-52.3509, 20.2181) -> (-52.3213, 20.2181) projected
  line L194 (-58.4938, 20.9097) -> (-58.8792, 20.9097) projected
  line L195 (-58.8792, 20.9097) -> (-58.8792, 19.2004) projected
  line L196 (-59.7906, 19.5858) -> (-59.7906, 20.9097) projected
  line L197 (-59.7906, 20.9097) -> (-60.1759, 20.9097) projected
  line L198 (-60.1759, 20.9097) -> (-60.1759, 19.403) projected
  line L199 (-61.0874, 19.5858) -> (-61.0874, 20.9097) projected
  line L200 (-61.0874, 20.9097) -> (-61.4727, 20.9097) projected
  line L201 (-61.4727, 20.9097) -> (-61.4727, 19.403) projected
  line L202 (-58.8792, 18.8744) -> (-58.8792, 18.6224) projected
  line L203 (-58.8792, 18.6224) -> (-58.4938, 18.6224) projected
  line L204 (-58.4938, 18.6224) -> (-58.4938, 20.9097) projected
  line L205 (-64.6738, 18.6224) -> (-64.2885, 18.6224) projected
  line L206 (-64.2885, 18.6224) -> (-64.2885, 20.9097) projected
  line L207 (-64.2885, 20.9097) -> (-64.6738, 20.9097) projected
  line L208 (-64.6738, 20.9097) -> (-64.6738, 19.2004) projected
  line L209 (-65.6989, 19.6055) -> (-65.6989, 20.9097) projected
  line L210 (-65.6989, 20.9097) -> (-66.0842, 20.9097) projected
  line L211 (-66.0842, 20.9097) -> (-66.0842, 19.4252) projected
  line L212 (-64.6738, 18.8769) -> (-64.6738, 18.6224) projected
  line L213 (-53.8885, 23.6632) -> (-53.9231, 23.6632) projected
  line L214 (-53.9231, 23.6632) -> (-53.9231, 23.1741) projected
  line L215 (-53.9354, 25.8121) -> (-53.9354, 24.4808) projected
  line L216 (-53.9354, 24.4808) -> (-52.8289, 24.4808) projected
  line L217 (-52.8289, 24.4808) -> (-52.8289, 24.8365) projected
  line L218 (-52.8289, 24.8365) -> (-53.5353, 24.8365) projected
  line L219 (-53.5353, 24.8365) -> (-53.5353, 25.6244) projected
  line L220 (-54.7999, 24.0683) -> (-54.7999, 23.7274) projected
  line L221 (-54.7999, 23.7274) -> (-54.4146, 23.7274) projected
  line L222 (-54.4146, 23.7274) -> (-54.4146, 26.0147) projected
  line L223 (-54.4146, 26.0147) -> (-54.7999, 26.0147) projected
  line L224 (-54.7999, 26.0147) -> (-54.7999, 24.3919) projected
  line L225 (-55.6076, 24.1399) -> (-55.6274, 24.1399) projected
  line L226 (-55.6274, 24.1399) -> (-55.6274, 23.7398) projected
  line L227 (-60.9231, 23.7274) -> (-60.5378, 23.7274) projected
  line L228 (-60.5378, 23.7274) -> (-60.5378, 26.0147) projected
  line L229 (-60.5378, 26.0147) -> (-60.9231, 26.0147) projected
  line L230 (-60.9231, 26.0147) -> (-60.9231, 24.3054) projected
  line L231 (-61.9482, 24.7105) -> (-61.9482, 26.0147) projected
  line L232 (-61.9482, 26.0147) -> (-62.3335, 26.0147) projected
  line L233 (-62.3335, 26.0147) -> (-62.3335, 24.5302) projected
  line L234 (-60.9231, 23.9818) -> (-60.9231, 23.7274) projected
  line L235 (-58.5692, 25.0316) -> (-58.5692, 23.7274) projected
  line L236 (-58.5692, 23.7274) -> (-58.1838, 23.7274) projected
  line L237 (-58.1838, 23.7274) -> (-58.1838, 25.2119) projected
  line L238 (-59.5942, 25.7627) -> (-59.5942, 26.0147) projected
  line L239 (-59.5942, 26.0147) -> (-59.9795, 26.0147) projected
  line L240 (-59.9795, 26.0147) -> (-59.9795, 23.7274) projected
  line L241 (-59.9795, 23.7274) -> (-59.5942, 23.7274) projected
  line L242 (-59.5942, 23.7274) -> (-59.5942, 25.4367) projected
  line L243 (49.0315, 22.2607) -> (50.1317, 22.8959) projected
  line L244 (48.4823, 19.0497) -> (49.163, 19.4427) projected
  line L245 (49.163, 19.4427) -> (49.1408, 19.4812) projected
  line L246 (48.3722, 21.8801) -> (48.5007, 21.9542) projected
  line L247 (50.6883, 23.2173) -> (51.1078, 23.4595) projected
  line L248 (51.1078, 23.4595) -> (50.7222, 24.1273) projected
  line L249 (50.7222, 24.1273) -> (48.0123, 22.5628) projected
  line L250 (-64.2477, 25.7825) -> (-64.2477, 26.0147) projected
  line L251 (-64.2477, 26.0147) -> (-64.6331, 26.0147) projected
  line L252 (-64.6331, 26.0147) -> (-64.6331, 22.8308) projected
  line L253 (-64.6331, 22.8308) -> (-64.2477, 22.8308) projected
  line L254 (-64.2477, 22.8308) -> (-64.2477, 23.8188) projected
  line L255 (-64.2477, 24.1374) -> (-64.2477, 25.4589) projected
  line L256 (48.2466, 24.8956) -> (46.3587, 23.8056) projected
  line L257 (46.3587, 23.8056) -> (45.6493, 25.0342) projected
  line L258 (45.6493, 25.0342) -> (45.0971, 24.7154) projected
  line L259 (45.0971, 24.7154) -> (45.8064, 23.4868) projected
  line L260 (45.8064, 23.4868) -> (44.6677, 22.8293) projected
  line L261 (44.6677, 22.8293) -> (45.0533, 22.1615) projected
  line L262 (45.0533, 22.1615) -> (46.192, 22.8189) projected
  line L263 (46.192, 22.8189) -> (46.4515, 22.3694) projected
  line L264 (46.4515, 22.3694) -> (47.0038, 22.6883) projected
  line L265 (47.0038, 22.6883) -> (46.7443, 23.1378) projected
  line L266 (46.7443, 23.1378) -> (48.9404, 24.4057) projected
  line L267 (49.027, 26.9844) -> (48.4277, 26.6383) projected
  line L268 (48.4277, 26.6383) -> (48.4499, 26.5998) projected
  line L269 (48.7342, 15.3707) -> (49.5424, 13.9708) projected
  line L270 (49.5424, 13.9708) -> (54.8251, 17.0208) projected
  line L271 (54.8251, 17.0208) -> (53.9502, 18.5363) projected
  line L272 (50.3906, 17.9196) -> (50.3649, 17.9048) projected
  line L273 (53.4917, 17.9463) -> (53.8204, 17.3769) projected
  line L274 (53.8204, 17.3769) -> (51.8683, 16.2498) projected
  line L275 (51.8683, 16.2498) -> (51.4086, 17.0461) projected
  line L276 (50.8221, 16.7075) -> (51.2818, 15.9112) projected
  line L277 (51.2818, 15.9112) -> (49.7364, 15.019) projected
  line L278 (49.7364, 15.019) -> (49.3483, 15.6911) projected
  line L279 (43.5091, 31.0249) -> (44.7178, 28.9315) projected
  line L280 (45.2272, 29.2257) -> (43.6429, 31.9698) projected
  line L281 (43.6429, 31.9698) -> (43.279, 31.7597) projected
  line L282 (45.3545, 32.8609) -> (44.6267, 32.4408) projected
  line L283 (44.6267, 32.4408) -> (44.649, 32.4022) projected
  line L284 (44.9548, 26.2372) -> (44.2454, 27.4659) projected
  line L285 (44.2454, 27.4659) -> (43.6932, 27.147) projected
  line L286 (43.6932, 27.147) -> (44.4025, 25.9184) projected
  line L287 (44.4025, 25.9184) -> (43.2638, 25.2609) projected
  line L288 (43.2638, 25.2609) -> (43.6494, 24.5931) projected
  line L289 (43.6494, 24.5931) -> (44.7881, 25.2505) projected
  line L290 (44.7881, 25.2505) -> (45.0476, 24.801) projected
  line L291 (45.0476, 24.801) -> (45.5999, 25.1199) projected
  line L292 (45.5999, 25.1199) -> (45.3404, 25.5694) projected
  line L293 (45.3404, 25.5694) -> (47.5365, 26.8373) projected
  line L294 (47.6231, 29.416) -> (47.0238, 29.0699) projected
  line L295 (47.0238, 29.0699) -> (47.046, 29.0314) projected
  line L296 (46.8427, 27.3272) -> (44.9548, 26.2372) projected
  line L297 (41.407, 32.4712) -> (40.8162, 32.1301) projected
  line L298 (40.8162, 32.1301) -> (41.2018, 31.4623) projected
  line L299 (41.2018, 31.4623) -> (45.166, 33.751) projected
  line L300 (45.166, 33.751) -> (44.7804, 34.4188) projected
  line L301 (44.7804, 34.4188) -> (41.9678, 32.795) projected
  line L302 (40.7229, 33.9427) -> (40.7031, 33.977) projected
  line L303 (40.7031, 33.977) -> (40.0096, 33.5766) projected
  line L304 (41.8523, 37.1177) -> (39.5408, 34.3391) projected
  line L305 (39.5408, 34.3391) -> (39.9561, 33.6199) projected
  line L306 (39.9561, 33.6199) -> (42.8972, 37.2358) projected
  line L307 (42.8972, 37.2358) -> (44.9599, 37.4792) projected
  line L308 (44.9599, 37.4792) -> (44.5472, 38.1941) projected
  line L309 (44.5472, 38.1941) -> (37.8922, 37.1945) projected
  line L310 (37.8922, 37.1945) -> (38.2927, 36.501) projected
  line L311 (38.2927, 36.501) -> (41.8523, 37.1177) projected
  circle A0 centre (-32.9006, 6.7452) radius 0.8 projected
  circle A1 centre (-32.9006, 31.2452) radius 0.8 projected
  circle A2 centre (62.7211, 7.3446) radius 1.25 projected
  circle A3 centre (50.2211, 28.9952) radius 1.25 projected
  circle A4 centre (37.7211, 50.6458) radius 1.25 projected
  circle A5 centre (-29, -42) radius 1.25 projected
  circle A6 centre (29, -90) radius 1.25 projected
  circle A7 centre (-29, -90) radius 1.25 projected
  circle A8 centre (29, -42) radius 1.25 projected
  circle A9 centre (30.0167, -0.0096) radius 2 projected
  circle A10 centre (15.0167, -25.9904) radius 2 projected
  circle A11 centre (50.8013, -12.0096) radius 2 projected
  circle A12 centre (35.8013, -37.9904) radius 2 projected
  circle A13 centre (-15.0167, -25.9904) radius 2 projected
  circle A14 centre (-30.0167, -0.0096) radius 2 projected
  circle A15 centre (-35.8013, -37.9904) radius 2 projected
  circle A16 centre (-50.8013, -12.0096) radius 2 projected
  circle A17 centre (-15, 26) radius 2 projected
  circle A18 centre (15, 50) radius 2 projected
  circle A19 centre (-15, 50) radius 2 projected
  circle A20 centre (15, 26) radius 2 projected
  circle A21 centre (0, 0) radius 15 projected
  circle A22 centre (0, 0) radius 100 projected
  circle A23 centre (15.0167, -25.9904) radius 2 construction
  line L312 (15.0167, -25.9904) -> (-15.0167, -25.9904) construction
  circle A24 centre (29, -42) radius 1.25 construction
  line L313 (29, -42) -> (-29, -42) construction
  line L314 (0, -42) -> (0, -25.9904) construction
  line L315 (-8, -23.9952) -> (8, -23.9952) construction
  line L316 (8, -23.9952) -> (8, -43.9952) construction
  line L317 (8, -43.9952) -> (-8, -43.9952) construction
  line L318 (-8, -43.9952) -> (-8, -23.9952) construction
  line L319 (-8, -23.9952) -> (8, -43.9952) construction
  line L320 (8, -23.9952) -> (-8, -43.9952) construction
  line L321 (8, -43.9952) -> (-8, -43.9952)
  line L322 (-8, -43.9952) -> (-8, -23.9952)
  line L323 (-8, -23.9952) -> (8, -23.9952)
  line L324 (8, -23.9952) -> (8, -43.9952)
  point P0 (0, -33.9952)
  dimension "d54" = 16
  dimension "d55" = 20
  constraints: 26 end point, 5 midpoint, 4 horizontal, 4 parallel, 2 perpendicular, 299 other
  measures "d54" distance of L316.end L317.end
  measures "d55" distance of L315.end L316.end
extrude "Extrusion2" cut sketch "Sketch7" against normal through all contours L321 L322 L323 L324